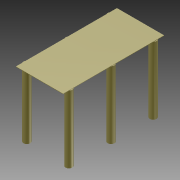
# Autodesk Inventor part: GP-terminals
Saved by Autodesk Inventor 2011 SP1 (Build 150282100, 282)
## iProperties
Created: 2013-12-24
Part Number: GP-terminals
Catalog Web Link: www.cadenas.de
Description: G Series - Ultra-Miniature Fully Illuminated Toggles - terminals-
Vendor: NKKSWITCHES
Document SubType Name: Modeling
Designer: PARTuser1
Manufacturer: NKKSWITCHES
Density: 1 g/cm^3
Category: PARTsolutions
Company: NKKSWITCHES
Title: GP-terminals
Author: Cadenas PARTsolutions
PSOL_IDENT_0: {$CADENAS_DATA\23d-libs\nkkswitches\toggle\g_ill\parts\g_ill_terminals.prj},230 {VTYP=3D},{NB=GP-ter
PSOL_IDENT_1: minals},{LINA=GP-terminals},{NN=G Series - Ultra-Miniature Fully Illuminated Toggles - terminals},{D
PSOL_IDENT_2: ATE=21.04.2009 08:12:26},{GEOMDATE=26.03.2009 08:32:00},{VERSION=},{LINEID=10},{LINESUBID=-1},{WBVAR
PSOL_IDENT_3: =TRMNLS}  {NB=GP-terminals},{LINA=GP-terminals},{KT=DUMMY},{PN=GP},{SRS=G},{TRMNLS=P}
CNS_NN: G Series - Ultra-Miniature Fully Illuminated Toggles - terminals
CNS_NB: GP-terminals
CNS_NBSYN: $PN.-terminals
CNS_LINA: GP-terminals
CNS_PN: GP
CNS_SRS: G
CNS_TRMNLS: P - Straight
SUPPLIER: NKKSWITCHES
ARTICLENO: GP-terminals
BOMINFO: GP-terminals
CREATOR: CADENAS GmbH
Autodesk Inventor part; units mm, degrees
sketch "Sketch_1" plane through (0, 0, 0) normal (0, 1, 0) x (-1, 0, 0)
  line L0 (1.4224, 3.048) -> (-1.4224, 3.048)
  line L1 (-1.4224, 3.048) -> (-1.4224, -3.048)
  line L2 (-1.4224, -3.048) -> (1.4224, -3.048)
  line L3 (1.4224, -3.048) -> (1.4224, 3.048)
  constraints: 8 end point
extrude "Extrusion1" add sketch "Sketch_1" along normal blind 0.0254
sketch "Sketch_2" plane through (0, 0, 0) normal (0, 1, 0) x (-1, 0, 0)
  circle A0 centre (-1.27, -2.54) radius 0.2032
  constraints: 1 centre point
extrude "Extrusion2" add sketch "Sketch_2" against normal blind 4.064
pattern_linear "Rectangular Pattern1" count 2 spacing 2.54 along (-1, 0, 0) count 3 spacing 2.54 along (0, 0, 1) of "Extrusion2"
ref_plane "to_body_XY" through (0, -0.9652, 0) normal (0, -1, 0) x (1, 0, 0)
ref_plane "to_body_YZ" through (0, -0.9652, 0) normal (1, 0, 0) x (0, 0, 1)
ref_plane "to_body_ZX" through (0, -0.9652, 0) normal (0, 0, 1) x (0, -1, 0)
body "Solid1"
